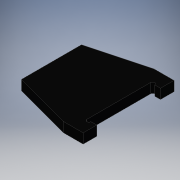
# Autodesk Inventor part: 胴体_サブフレーム_1_7
Saved by Autodesk Inventor 2018 (Build 220112000, 112)
## iProperties
Created: 2016-05-15
Part Number: 胴体_サブフレーム_1_7
Material: アセタール樹脂、黒
Document SubType Name: Modeling
Designer: hiroaki
Density: 1.425 g/cm^3
Appearance: 滑らか - 黒
Mass: 6.61533 g
Surface Area: 42.3195 cm^2
Volume: 4.64234 cm^3
Author: hiroaki
Autodesk Inventor part; units mm, degrees
ref_plane "YZ Plane" through (0, 0, 0) normal (1, 0, 0) x (0, 1, 0)
ref_plane "XZ Plane" through (0, 0, 0) normal (0, 1, 0) x (-1, 0, 0)
ref_plane "XY Plane" through (0, 0, 0) normal (0, 0, 1) x (1, 0, 0)
sketch "スケッチ1" plane through (0, 0, 0) normal (0, 0, 1) x (1, 0, 0)
  line L0 (0, 16.25) -> (28.4656, 16.25) construction
  line L1 (28.4656, 16.25) -> (28.4656, -16.25) construction
  line L2 (28.4656, -16.25) -> (0, -16.25) construction
  line L3 (0, -16.25) -> (0, 16.25) construction
  line L4 (5, 23.25) -> (-5.1583, 23.25)
  line L5 (-5.1583, 23.25) -> (-34.5, 15.3879)
  line L6 (-34.5, 15.3879) -> (-34.5, -15.3879)
  line L7 (-34.5, -15.3879) -> (-5.1583, -23.25)
  line L8 (-5.1583, -23.25) -> (5, -23.25)
  line L9 (5, -23.25) -> (5, -16.3)
  line L10 (5, -16.3) -> (2.05, -16.3)
  arc A0 (-0.05, -16.3) -> (2.05, -16.3) centre (1, -16.3) ccw
  line L11 (-0.05, -16.3) -> (-0.05, 16.3)
  arc A1 (2.05, 16.3) -> (-0.05, 16.3) centre (1, 16.3) ccw
  line L12 (28.4656, 0) -> (0, 0) construction
  line L13 (2.05, 16.3) -> (5, 16.3)
  line L14 (5, 16.3) -> (5, 23.25)
  line L15 (28.5156, 16.3) -> (-0.05, 16.3) construction
  line L16 (-0.05, 16.3) -> (-0.05, -16.3) construction
  line L17 (-0.05, -16.3) -> (28.5156, -16.3) construction
  line L18 (28.5156, -16.3) -> (28.5156, 16.3) construction
  circle A2 centre (-4.5, 18.25) radius 1.2
  circle A3 centre (-4.5, -18.25) radius 1.2
  line L19 (0, 0) -> (28.4656, 0) construction
  line L20 (2.5, 16.25) -> (2.5, -16.25) construction
  circle A4 centre (-4.5, 18.25) radius 5 construction
  line L21 (-6.0877, 15.5) -> (-7.6754, 18.25)
  line L22 (-7.6754, 18.25) -> (-6.0877, 21)
  line L23 (-6.0877, 21) -> (-2.9123, 21)
  line L24 (-2.9123, 21) -> (-1.3246, 18.25)
  line L25 (-1.3246, 18.25) -> (-2.9123, 15.5)
  line L26 (-2.9123, 15.5) -> (-6.0877, 15.5)
  point P0 (-34.5, 0)
  point P1 (-0.05, 0)
  dimension "d98" = 32.5
  dimension "d100" = 0.05
  dimension "d101" = 1.05
  dimension "d102" = 5
  dimension "d104" = 2.4
  dimension "d106" = 2.5
  dimension "d107" = 7
  dimension "d108" = 18.25
  dimension "d109" = 5
  dimension "d110" = 30
  dimension "d111" = 165
  dimension "d130" = 5.5
  constraints: 54 end point, 6 equal length, 5 centre point, 4 coincident, 4 horizontal, 4 midpoint, 4 perpendicular, 4 point on circle, 4 point on line, 4 tangent, 3 collinear, 3 symmetric about line, 3 vertical, 2 equal radius, 1 horizontal alignment, 1 vertical alignment, 17 other
  measures "d98" distance of L0.end L1.end
  measures "d100" distance between parallel lines of L0 L15
  measures "d101" radius of A0
  measures "d102" distance between parallel lines of L14 L3
  measures "d104" diameter of A2
  measures "d106" distance between parallel lines of L20 L3
  measures "d107" distance from line of A2.centre L20
  measures "d108" distance from line of L12 A2.centre
  measures "d109" distance from line of A2.centre L4
  measures "d110" distance from line of A2.centre L6
  measures "d111" angle of L4 L5
  measures "d130" distance between parallel lines of L26 L23
extrude "押し出し1" add sketch "スケッチ1" along normal blind 5 contours L14 L13 A1 L11 A0 L10 L9 L8 L7 L6 L5 L4 | L21 L22 L23 L24 L25 L26
sketch "スケッチ8" plane through (0, 0, 0) normal (0, 0, -1) x (-1, 0, 0)
  circle A0 centre (4.5, 18.25) radius 1.2 projected
  circle A1 centre (4.5, 18.25) radius 1.2
  circle A2 centre (4.5, -18.25) radius 1.2 projected
  circle A3 centre (4.5, -18.25) radius 1.2
  point P0 (0, 0)
  constraints: 2 centre point, 2 coincident
extrude "押し出し6" add sketch "スケッチ8" against normal up to surface (5 mm away)
